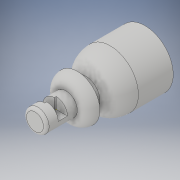
# Autodesk Inventor part: Elektrodenhalter_final_big_withCableCanal
Saved by Autodesk Inventor 2018 (Build 220112000, 112)
## iProperties
Part Number: Elektrodenhalter_final_big_withCableCanal
Material: Generisch
Document SubType Name: Modeling
Designer: Timo
Density: 1 g/cm^3
Appearance: Vorgabe
Author: Timo
Autodesk Inventor part; units mm, degrees
ref_plane "YZ Plane" through (0, 0, 0) normal (1, 0, 0) x (0, 1, 0)
ref_plane "XZ Plane" through (0, 0, 0) normal (0, 1, 0) x (-1, 0, 0)
ref_plane "XY Plane" through (0, 0, 0) normal (0, 0, 1) x (1, 0, 0)
sketch "Skizze1" plane through (0, 0, 0) normal (0, 1, 0) x (-1, 0, 0)
  circle A0 centre (0, 0) radius 4
  dimension "d0" = 8
  constraints: 1 centre point, 1 coincident
  measures "d0" diameter of A0
extrude "Extrusion1" add sketch "Skizze1" along normal blind 2
fillet "Rundung1" radius 2 1 edges at (4, 0, 0)
sketch "Skizze2" plane through (0, 2, 0) normal (0, 1, 0) x (1, 0, 0)
  circle A0 centre (0, 0) radius 2.5
  dimension "d4" = 5
  constraints: 1 centre point, 1 coincident
  measures "d4" diameter of A0
extrude "Extrusion2" add sketch "Skizze2" along normal blind 1.5
sketch "Skizze3" plane through (0, 3.5, 0) normal (0, 1, 0) x (1, 0, 0)
  circle A0 centre (0, 0) radius 5
  dimension "d7" = 10
  constraints: 1 centre point, 1 coincident
  measures "d7" diameter of A0
extrude "Extrusion3" add sketch "Skizze3" along normal blind 8
sketch "Skizze5" plane through (0, 11.5, 0) normal (0, 1, 0) x (1, 0, 0)
  circle A0 centre (0, 0) radius 5
  dimension "d13" = 10
  constraints: 1 centre point, 1 coincident
  measures "d13" diameter of A0
extrude "Extrusion5" add sketch "Skizze5" along normal blind 2.5
sketch "Skizze6" plane through (0, 14, 0) normal (0, 1, 0) x (1, 0, 0)
  circle A0 centre (0, 0) radius 4.25
  dimension "d16" = 8.5
  constraints: 1 centre point, 1 coincident
  measures "d16" diameter of A0
extrude "Extrusion6" cut sketch "Skizze6" against normal blind 2.5
sketch "Skizze8" plane through (0, 11.5, 0) normal (0, 1, 0) x (1, 0, 0)
  circle A0 centre (0, 0) radius 0.8
  dimension "d19" = 1.6
  constraints: 1 centre point, 1 coincident
  measures "d19" diameter of A0
extrude "Extrusion7" add sketch "Skizze8" along normal blind 1.6
fillet "Rundung2" radius 5 1 edges at (-5, 3.5, 0)
sketch "Skizze13" plane through (0, 0, 0) normal (0, -1, 0) x (1, 0, 0)
  circle A0 centre (0, 0) radius 2
  dimension "d26" = 4
  constraints: 1 centre point, 1 coincident
  measures "d26" diameter of A0
extrude "Extrusion9" add sketch "Skizze13" along normal blind 1.75 separate body
sketch "Skizze16" plane through (0, -1.75, 0) normal (0, -1, 0) x (1, 0, 0)
  circle A0 centre (0, 0) radius 2
  circle A1 centre (0, 0) radius 2 projected
  line L0 (-2, 0) -> (2, 0)
  dimension "d35" = 4
  constraints: 2 end point, 2 point on circle, 1 centre point, 1 coincident, 1 horizontal
  measures "d35" diameter of A0
extrude "Extrusion12" add sketch "Skizze16" along normal blind 2 contours A0 L0 picked at (-0.5903, -0.3098) bodies 2
sketch "Skizze17" plane through (0, -3.75, 0) normal (0, -1, 0) x (1, 0, 0)
  circle A0 centre (0, 0) radius 2
  dimension "d38" = 4
  constraints: 1 centre point, 1 coincident
  measures "d38" diameter of A0
extrude "Extrusion13" add sketch "Skizze17" along normal blind 1.75 bodies 2
sketch "Skizze19" plane through (0, -1.75, 0) normal (0, -1, 0) x (1, 0, 0)
  point P0 (0, 0)
sketch "Skizze20" plane through (0, -1.75, 0) normal (0, -1, 0) x (1, 0, 0)
  point P0 (0, 0)
sketch "Skizze21" plane through (0, -1.75, 0) normal (0, -1, 0) x (1, 0, 0)
  point P0 (0, 0)
sketch "Skizze22" plane through (0, -1.75, 0) normal (0, -1, 0) x (1, 0, 0)
  point P0 (0, 0)
sketch "Skizze24" plane through (0, -3.75, 0) normal (0, 1, 0) x (1, 0, 0)
  point P0 (0, 0)
sketch "Skizze28" plane through (0, -1.75, 0) normal (0, -1, 0) x (1, 0, 0)
  circle A0 centre (0, 0) radius 2
  line L0 (0, 2) -> (0, 0)
  line L1 (-2, 0) -> (2, 0) projected
  line L2 (0, 0) -> (-2, 0)
  dimension "d51" = 4
  constraints: 4 end point, 1 centre point, 1 coincident, 1 collinear, 1 point on circle, 1 vertical
  measures "d51" diameter of A0
extrude "Extrusion15" add sketch "Skizze28" along normal blind 0.35 contours L0 L1 A0 picked at (-1.3166, 0.1483) bodies 2
sketch "Skizze32" plane through (0, -3.75, 0) normal (0, 1, 0) x (1, 0, 0)
  circle A0 centre (0, 0) radius 2
  line L0 (0, 0) -> (2, 0) projected
  line L1 (0, 0) -> (0, -2) projected
  line L2 (0, 0) -> (0, -2)
  line L3 (0, 0) -> (2, 0)
  dimension "d55" = 4
  constraints: 4 end point, 2 collinear, 1 centre point, 1 coincident
  measures "d55" diameter of A0
extrude "Extrusion16" add sketch "Skizze32" along normal blind 0.35 contours A0 L1 L0 picked at (1.3166, -0.1483) bodies 2
fillet "Rundung4" radius 0.5 1 edges at (-2, -5.5, 0)
